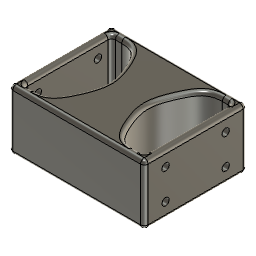
5717bfef-9a5b-4853-904e-d138bfb05230 (Autodesk Fusion 360 design; units mm, degrees)
part number: 2026-05-17-06-05-02-434
Autodesk Fusion 360 part; units mm, degrees
note: some values were not read from the file. Set by a fixed rule: which sketch regions a step uses.
sketch "スケッチ1" plane through (0, 0, 0) normal (0, 0, 1) x (1, 0, 0)
  line L0 (1.5, 0) -> (52.5, 0)
  line L1 (54, 1.5) -> (54, 39.5)
  line L2 (52.5, 41) -> (1.5, 41)
  line L3 (0, 39.5) -> (0, 1.5)
  arc A0 (1.5, 41) -> (0, 39.5) centre (1.5, 39.5) ccw
  arc A1 (0, 1.5) -> (1.5, 0) centre (1.5, 1.5) ccw
  arc A2 (54, 39.5) -> (52.5, 41) centre (52.5, 39.5) ccw
  arc A3 (52.5, 0) -> (54, 1.5) centre (52.5, 1.5) ccw
  point P0 (54, 0)
  point P1 (0, 41)
  dimension "d1" = 54
  dimension "d2" = 41
  dimension "d7" = 1.5
  dimension "d8" = 1.5
  dimension "d9" = 1.5
  constraint horizontal L0
  constraint vertical L1
  constraint horizontal L2
  constraint vertical L3
  constraint coincident P1 L2
  constraint coincident P1 L3
  constraint tangent L2 A0
  constraint tangent L3 A0
  constraint coincident origin L0
  constraint coincident origin L3
  constraint tangent L0 A1
  constraint tangent L3 A1
  constraint tangent L1 A2
  constraint tangent L2 A2
  constraint coincident P0 L0
  constraint coincident P0 L1
  constraint tangent L0 A3
  constraint tangent L1 A3
  constraint equal A2 A3
  measures "d1" distance of origin P0
  measures "d2" distance of origin P1
  measures "d7" radius of A0
  measures "d8" radius of A1
  measures "d9" radius of A2
extrude "押し出し1" add sketch "スケッチ1" along normal blind 24
sketch "スケッチ2" plane through (0, 0, 24) normal (0, 0, 1) x (-1, 0, 0)
  line L0 (0, -39.5) -> (0, -1.5)
  line L1 (-1.5, 0) -> (-52.5, 0)
  line L2 (-54, -1.5) -> (-54, -39.5)
  line L3 (-52.5, -41) -> (-1.5, -41)
  arc A0 (-52.5, 0) -> (-54, -1.5) centre (-52.5, -1.5) ccw
  arc A1 (-54, -39.5) -> (-52.5, -41) centre (-52.5, -39.5) ccw
  arc A2 (-1.5, -41) -> (0, -39.5) centre (-1.5, -39.5) ccw
  arc A3 (0, -1.5) -> (-1.5, 0) centre (-1.5, -1.5) ccw
  line L4 (-4.5, -3) -> (-49.5, -3)
  line L5 (-51, -4.5) -> (-51, -36.5)
  line L6 (-49.5, -38) -> (-4.5, -38)
  line L7 (-3, -36.5) -> (-3, -4.5)
  arc A4 (-4.5, -38) -> (-3, -36.5) centre (-4.5, -36.5) ccw
  arc A5 (-3, -4.5) -> (-4.5, -3) centre (-4.5, -4.5) ccw
  arc A6 (-51, -36.5) -> (-49.5, -38) centre (-49.5, -36.5) ccw
  arc A7 (-49.5, -3) -> (-51, -4.5) centre (-49.5, -4.5) ccw
  spline S0 degree 5 poles (-7, -38) (-7.5583, -38) (-8.6151, -37.9499) (-10.0214, -37.7246) (-11.5634, -37.1267) (-13.0719, -35.9068) (-14.322, -34.2589) (-15.4541, -32.2503) (-16.5315, -29.9805) (-17.5227, -27.5722) (-18.3465, -25.1441) (-18.9011, -22.7752) (-19.0986, -20.5) (-18.8989, -18.2248) (-18.3435, -15.8559) (-17.5199, -13.4278) (-16.5299, -11.0195) (-15.4539, -8.7497) (-14.3226, -6.7411) (-13.0727, -5.0932) (-11.5639, -3.8733) (-10.0216, -3.2754) (-8.6151, -3.0501) (-7.5583, -3) (-7, -3) knots 0 0 0 0 0 0 0.05 0.1 0.15 0.2 0.25 0.3 0.35 0.4 0.45 0.5 0.55 0.6 0.65 0.7 0.75 0.8 0.85 0.9 0.95 1 1 1 1 1 1
  line L8 (-19.0016, -24.1157) -> (-18.9984, -16.8843)
  line L9 (-2, -38) -> (-12, -38)
  line L10 (-12, -3) -> (-2, -3)
  spline S1 degree 5 poles (-7, -38) (-7.5583, -38) (-8.6151, -37.9499) (-10.0214, -37.7246) (-11.5634, -37.1267) (-13.0719, -35.9068) (-14.322, -34.2589) (-15.4541, -32.2503) (-16.5315, -29.9805) (-17.5227, -27.5722) (-18.3465, -25.1441) (-18.9011, -22.7752) (-19.0986, -20.5) (-18.8989, -18.2248) (-18.3435, -15.8559) (-17.5199, -13.4278) (-16.5299, -11.0195) (-15.4539, -8.7497) (-14.3226, -6.7411) (-13.0727, -5.0932) (-11.5639, -3.8733) (-10.0216, -3.2754) (-8.6151, -3.0501) (-7.5583, -3) (-7, -3) knots 0 0 0 0 0 0 0.05 0.1 0.15 0.2 0.25 0.3 0.35 0.4 0.45 0.5 0.55 0.6 0.65 0.7 0.75 0.8 0.85 0.9 0.95 1 1 1 1 1 1
  line L11 (-2, -38) -> (-12, -38)
  line L12 (-19.0016, -24.1157) -> (-18.9984, -16.8843)
  line L13 (-12, -3) -> (-2, -3)
  spline S2 degree 5 poles (-7, -38) (-7.5583, -38) (-8.6151, -37.9499) (-10.0214, -37.7246) (-11.5634, -37.1267) (-13.0719, -35.9068) (-14.322, -34.2589) (-15.4541, -32.2503) (-16.5315, -29.9805) (-17.5227, -27.5722) (-18.3465, -25.1441) (-18.9011, -22.7752) (-19.0986, -20.5) (-18.8989, -18.2248) (-18.3435, -15.8559) (-17.5199, -13.4278) (-16.5299, -11.0195) (-15.4539, -8.7497) (-14.3226, -6.7411) (-13.0727, -5.0932) (-11.5639, -3.8733) (-10.0216, -3.2754) (-8.6151, -3.0501) (-7.5583, -3) (-7, -3) knots 0 0 0 0 0 0 0.05 0.1 0.15 0.2 0.25 0.3 0.35 0.4 0.45 0.5 0.55 0.6 0.65 0.7 0.75 0.8 0.85 0.9 0.95 1 1 1 1 1 1
  line L14 (-2, -38) -> (-12, -38)
  line L15 (-19.0016, -24.1157) -> (-18.9984, -16.8843)
  line L16 (-12, -3) -> (-2, -3)
  spline S3 degree 5 poles (-7, -38) (-7.5583, -38) (-8.6151, -37.9499) (-10.0214, -37.7246) (-11.5634, -37.1267) (-13.0719, -35.9068) (-14.322, -34.2589) (-15.4541, -32.2503) (-16.5315, -29.9805) (-17.5227, -27.5722) (-18.3465, -25.1441) (-18.9011, -22.7752) (-19.0986, -20.5) (-18.8989, -18.2248) (-18.3435, -15.8559) (-17.5199, -13.4278) (-16.5299, -11.0195) (-15.4539, -8.7497) (-14.3226, -6.7411) (-13.0727, -5.0932) (-11.5639, -3.8733) (-10.0216, -3.2754) (-8.6151, -3.0501) (-7.5583, -3) (-7, -3) knots 0 0 0 0 0 0 0.05 0.1 0.15 0.2 0.25 0.3 0.35 0.4 0.45 0.5 0.55 0.6 0.65 0.7 0.75 0.8 0.85 0.9 0.95 1 1 1 1 1 1
  line L17 (-2, -38) -> (-12, -38)
  line L18 (-19.0016, -24.1157) -> (-18.9984, -16.8843)
  line L19 (-12, -3) -> (-2, -3)
  spline S4 degree 5 poles (-47.1875, -38) (-46.6247, -38.0005) (-45.5578, -37.9521) (-44.1334, -37.7314) (-42.5624, -37.1429) (-41.0158, -35.9379) (-39.7326, -34.304) (-38.5778, -32.3054) (-37.4884, -30.0394) (-36.4923, -27.6293) (-35.6661, -25.1955) (-35.1076, -22.8198) (-34.9018, -20.5391) (-35.0917, -18.2616) (-35.6402, -15.8896) (-36.46, -13.4569) (-37.4492, -11.0423) (-38.5257, -8.7653) (-39.6574, -6.7493) (-40.907, -5.0948) (-42.4155, -3.8695) (-43.9584, -3.2682) (-45.3665, -3.0409) (-46.4251, -2.9898) (-46.9843, -2.9893) knots 0 0 0 0 0 0 0.05 0.1 0.15 0.2 0.25 0.3 0.35 0.4 0.45 0.5 0.55 0.6 0.65 0.7 0.75 0.8 0.85 0.9 0.95 1 1 1 1 1 1
  line L20 (-52.1875, -37.9955) -> (-42.1875, -38.0045)
  line L21 (-35.0016, -24.1157) -> (-34.9984, -16.8843)
  line L22 (-41.9843, -2.9937) -> (-51.9843, -2.9848)
  point P0 (-15, -33)
  point P1 (-19, -20.5)
  point P2 (-15, -8)
  point P3 (-15, -33)
  point P4 (-19, -20.5)
  point P5 (-15, -8)
  point P6 (-15, -33)
  point P7 (-19, -20.5)
  point P8 (-15, -8)
  point P9 (-15, -33)
  point P10 (-19, -20.5)
  point P11 (-15, -8)
  point P12 (-35, -20.5)
  point P13 (-38.9888, -7.9964)
  point P14 (-39.0112, -32.9964)
  dimension "d10" = 3
  dimension "d11" = 3
  dimension "d12" = 3
  dimension "d13" = 3
  dimension "d14" = 1.5
  dimension "d15" = 1.5
  dimension "d16" = 1.5
  dimension "d17" = 1.5
  dimension "d18" = 17.5
  dimension "d19" = 16
  constraint horizontal L4
  constraint vertical L5
  constraint horizontal L6
  constraint vertical L7
  constraint tangent L6 A4
  constraint tangent L7 A4
  constraint tangent L4 A5
  constraint tangent L7 A5
  constraint tangent L5 A6
  constraint tangent L6 A6
  constraint tangent L4 A7
  constraint tangent L5 A7
  constraint coincident L6 S0.start
  constraint coincident L4 S0.end
  constraint midpoint P10 L8
  constraint midpoint S0.start L9
  constraint coincident L6 L9.start
  constraint midpoint S0.end L10
  constraint coincident L4 L10.end
  constraint midpoint P10 L12
  constraint midpoint S0.start L11
  constraint midpoint S0.end L13
  constraint midpoint P10 L15
  constraint midpoint S0.start L14
  constraint midpoint S0.end L16
  constraint coincident P10 P7
  constraint midpoint P10 L18
  constraint midpoint S0.start L17
  constraint midpoint S0.end L19
  constraint midpoint P12 L21
  constraint midpoint S4.start L20
  constraint midpoint S4.end L22
  constraint coincident L6 S4.start
  measures "d10" distance of L0 L7
  measures "d11" distance of L2 L5
  measures "d12" distance of L3 L6
  measures "d13" distance of L1 L4
  measures "d14" radius of A4
  measures "d15" radius of A5
  measures "d16" radius of A6
  measures "d17" radius of A7
  measures "d18" distance of L6 P10
  measures "d19" distance of L7 P10
extrude "押し出し2" cut sketch "スケッチ2" against normal up to surface (24 mm away) contours L4 L6 L7 A4 A5 S0 L9 L10 S1 L11 L13 S2 L14 L16 S3 L17 L19 | L4 L5 A6 A7 S4 L20 | L6 A6 L20
fillet "フィレット1" radius 1.5 8 edges at (27, 41, 24) (0.4393, 40.5607, 24) (0, 20.5, 24) (0.4393, 0.4393, 24) (27, 0, 24) (53.5607, 0.4393, 24) (54, 20.5, 24) (53.5607, 40.5607, 24)
fillet "フィレット2" radius 1.5 8 edges at (0, 20.5, 0) (0.4393, 0.4393, 0) (27, 0, 0) (53.5607, 0.4393, 0) (54, 20.5, 0) (53.5607, 40.5607, 0) (27, 41, 0) (0.4393, 40.5607, 0)
fillet "フィレット3" radius 1.5 6 edges at (35.0026, 20.7617, 24) (48.3324, 38, 24) (50.5607, 37.5607, 24) (51, 20.5, 24) (50.5607, 3.4393, 24) (47.9658, 3, 24)
fillet "フィレット4" radius 1.5 6 edges at (3.4393, 3.4393, 24) (3, 20.5, 24) (3.4393, 37.5607, 24) (5.75, 38, 24) (19, 20.5, 24) (5.75, 3, 24)
fillet "フィレット5" radius 1.5 6 edges at (47.9658, 3, 0) (50.5607, 3.4393, 0) (51, 20.5, 0) (50.5607, 37.5607, 0) (48.3324, 38, 0) (35.0026, 20.7617, 0)
fillet "フィレット6" radius 1.5 6 edges at (5.75, 3, 0) (19, 20.5, 0) (5.75, 38, 0) (3.4393, 37.5607, 0) (3, 20.5, 0) (3.4393, 3.4393, 0)
sketch "スケッチ3" plane through (0, 0, 0) normal (-1, 0, 0) x (0, -1, 0)
  line L0 (-39.5, 1.5) -> (-1.5, 1.5)
  line L1 (-1.5, 1.5) -> (-1.5, 22.5)
  line L2 (-1.5, 22.5) -> (-39.5, 22.5)
  line L3 (-39.5, 22.5) -> (-39.5, 1.5)
  circle A0 centre (-32.5, 18) radius 1.45
  circle A1 centre (-8.5, 6) radius 1.45
  circle A2 centre (-32.5, 6) radius 1.45
  circle A3 centre (-8.5, 18) radius 1.45
  line L4 (-1.5, 24) -> (-39.5, 24)
  line L5 (-39.5, 0) -> (-1.5, 0)
  dimension "d34" = 2.9
  dimension "d35" = 2.9
  dimension "d36" = 2.9
  dimension "d37" = 2.9
  dimension "d38" = 7
  dimension "d39" = 7
  dimension "d40" = 7
  dimension "d41" = 7
  dimension "d42" = 6
  dimension "d43" = 6
  dimension "d44" = 6
  dimension "d45" = 6
  measures "d34" diameter of A0
  measures "d35" diameter of A1
  measures "d36" diameter of A2
  measures "d37" diameter of A3
  measures "d38" distance of L3 A0.centre
  measures "d39" distance of L3 A2.centre
  measures "d40" distance of L1 A3.centre
  measures "d41" distance of L1 A1.centre
  measures "d42" distance of A0.centre L4
  measures "d43" distance of A2.centre L5
  measures "d44" distance of A3.centre L4
  measures "d45" distance of A1.centre L5
sketch "スケッチ4" plane through (54, 0, 0) normal (1, 0, 0) x (0, 1, 0)
  line L0 (1.5, 1.5) -> (39.5, 1.5)
  line L1 (39.5, 1.5) -> (39.5, 22.5)
  line L2 (39.5, 22.5) -> (1.5, 22.5)
  line L3 (1.5, 22.5) -> (1.5, 1.5)
  circle A0 centre (8.5, 18) radius 1.45
  circle A1 centre (8.5, 6) radius 1.45
  circle A2 centre (32.5, 18) radius 1.45
  circle A3 centre (32.5, 6) radius 1.45
  line L4 (1.5, 24) -> (39.5, 24)
  line L5 (39.5, 0) -> (1.5, 0)
  dimension "d46" = 2.9
  dimension "d47" = 2.9
  dimension "d48" = 2.9
  dimension "d49" = 2.9
  dimension "d50" = 7
  dimension "d51" = 7
  dimension "d52" = 7
  dimension "d53" = 7
  dimension "d54" = 6
  dimension "d55" = 6
  dimension "d56" = 6
  dimension "d57" = 6
  measures "d46" diameter of A0
  measures "d47" diameter of A1
  measures "d48" diameter of A2
  measures "d49" diameter of A3
  measures "d50" distance of L3 A0.centre
  measures "d51" distance of L3 A1.centre
  measures "d52" distance of L1 A3.centre
  measures "d53" distance of L1 A2.centre
  measures "d54" distance of A0.centre L4
  measures "d55" distance of A1.centre L5
  measures "d56" distance of A2.centre L4
  measures "d57" distance of A3.centre L5
extrude "押し出し3" cut sketch "スケッチ4" against normal up to surface (3 mm away) contours A0 | A1 | A2 | A3
extrude "押し出し4" cut sketch "スケッチ3" against normal up to surface (3 mm away) contours A0 | A1 | A2 | A3
equation "d18 = ( 35 / 2 ) * 1 mm"
equation "d39 = d38"
equation "d40 = d38"
equation "d41 = d38"
equation "d43 = d42"
equation "d44 = d42"
equation "d45 = d42"
equation "d51 = d50"
equation "d52 = d50"
equation "d53 = d50"
equation "d55 = d54"
equation "d56 = d54"
equation "d57 = d54"
